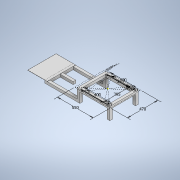
# Autodesk Inventor part: test1
Saved by Autodesk Inventor 2021 (Build 250183000, 183)
## iProperties
Created: 2023-12-08
Part Number: test1
Material: Generic
Document SubType Name: Modeling
Designer: assman
Density: 1 g/cm^3
Appearance: Default
Author: assman
Autodesk Inventor part; units mm, degrees
ref_plane "YZ Plane" through (0, 0, 0) normal (1, 0, 0) x (0, 1, 0)
ref_plane "XZ Plane" through (0, 0, 0) normal (0, 1, 0) x (-1, 0, 0)
ref_plane "XY Plane" through (0, 0, 0) normal (0, 0, 1) x (1, 0, 0)
sketch "Sketch1" plane through (0, 0, 0) normal (0, 1, 0) x (-1, 0, 0)
  line L0 (142.5, 197.5) -> (-142.5, 197.5) construction
  line L1 (-142.5, 197.5) -> (-142.5, -197.5) construction
  line L2 (-142.5, -197.5) -> (142.5, -197.5) construction
  line L3 (142.5, -197.5) -> (142.5, 197.5) construction
  line L4 (142.5, 197.5) -> (-142.5, -197.5) construction
  line L5 (-142.5, 197.5) -> (142.5, -197.5) construction
  line L6 (275, -235) -> (-275, -235) construction
  line L7 (-275, -235) -> (-275, 235) construction
  line L8 (-275, 235) -> (275, 235) construction
  line L9 (275, 235) -> (275, -235) construction
  line L10 (275, -235) -> (-275, 235) construction
  line L11 (-275, -235) -> (275, 235) construction
  line L12 (274.0052, -241.4689) -> (274.0052, -478.1407) construction
  line L13 (274.0052, -478.1407) -> (222.5538, -478.1407) construction
  line L14 (222.5538, -478.1407) -> (222.5538, -241.4689) construction
  line L15 (222.5538, -241.4689) -> (274.0052, -241.4689) construction
  line L16 (200, 212.5) -> (-200, 212.5)
  line L17 (-200, 212.5) -> (-200, 182.5)
  line L18 (-200, 182.5) -> (200, 182.5)
  line L19 (200, 182.5) -> (200, 212.5)
  line L20 (200, 212.5) -> (-200, 182.5) construction
  line L21 (-200, 212.5) -> (200, 182.5) construction
  line L22 (200, -182.5) -> (-200, -182.5)
  line L23 (-200, -182.5) -> (-200, -212.5)
  line L24 (-200, -212.5) -> (200, -212.5)
  line L25 (200, -212.5) -> (200, -182.5)
  line L26 (200, -182.5) -> (-200, -212.5) construction
  line L27 (-200, -182.5) -> (200, -212.5) construction
  circle A0 centre (142.5, 197.5) radius 4
  circle A1 centre (142.5, -197.5) radius 4
  circle A2 centre (-142.5, 197.5) radius 4
  circle A3 centre (-142.5, -197.5) radius 4
  point P0 (0, 0)
  point P1 (0, 197.5)
  point P2 (0, -197.5)
  dimension "d0" = 285
  dimension "d1" = 395
  dimension "d2" = 550
  dimension "d3" = 470
  dimension "d10" = 400
  dimension "d11" = 30
  dimension "d12" = 400
  dimension "d13" = 30
  dimension "d14" = 8
  dimension "d15" = 8
  dimension "d16" = 8
  dimension "d17" = 8
  constraints: 48 end point, 10 midpoint, 8 parallel, 4 centre point, 4 coincident, 4 horizontal, 4 perpendicular, 2 other
  measures "d0" distance of L2.end L1.end
  measures "d1" distance of L1.end L0.end
  measures "d2" distance of L7.end L8.end
  measures "d3" distance of L6.end L7.end
  measures "d10" distance of L18.end L17.end
  measures "d11" distance of L17.end L16.end
  measures "d12" distance of L24.end L23.end
  measures "d13" distance of L23.end L22.end
  measures "d14" diameter of A0
  measures "d15" diameter of A1
  measures "d16" diameter of A2
  measures "d17" diameter of A3
sketch "Sketch2" plane through (0, 0, 0) normal (0, 1, 0) x (-1, 0, 0)
  line L0 (142.5, 197.5) -> (-142.5, 197.5) construction
  line L1 (142.5, -197.5) -> (142.5, 197.5) construction
  line L2 (-142.5, -197.5) -> (142.5, -197.5) construction
  line L3 (-142.5, 197.5) -> (-142.5, -197.5) construction
  line L4 (250, 217.5) -> (-250, 217.5)
  line L5 (-250, 217.5) -> (-250, 177.5)
  line L6 (-250, 177.5) -> (250, 177.5)
  line L7 (250, 177.5) -> (250, 217.5)
  line L8 (250, 217.5) -> (-250, 177.5) construction
  line L9 (-250, 217.5) -> (250, 177.5) construction
  line L10 (250, -177.5) -> (-250, -177.5)
  line L11 (-250, -177.5) -> (-250, -217.5)
  line L12 (-250, -217.5) -> (250, -217.5)
  line L13 (250, -217.5) -> (250, -177.5)
  line L14 (250, -177.5) -> (-250, -217.5) construction
  line L15 (-250, -177.5) -> (250, -217.5) construction
  line L16 (250, 217.5) -> (210, 217.5)
  line L17 (210, 217.5) -> (210, -217.5)
  line L18 (210, -217.5) -> (250, -217.5)
  line L19 (250, -217.5) -> (250, 217.5)
  line L20 (-250, 217.5) -> (-210, 217.5)
  line L21 (-210, 217.5) -> (-210, -217.5)
  line L22 (-210, -217.5) -> (-250, -217.5)
  line L23 (-250, -217.5) -> (-250, 217.5)
  point P0 (0, 0)
  point P1 (0, 197.5)
  point P2 (0, -197.5)
  point P3 (210, -177.5)
  point P4 (-210, -177.5)
  point P5 (-210, 177.5)
  point P6 (210, 177.5)
  dimension "d4" = 500
  dimension "d5" = 40
  dimension "d6" = 500
  dimension "d7" = 40
  dimension "d8" = 40
  dimension "d9" = 40
  constraints: 40 end point, 8 parallel, 6 midpoint, 4 horizontal, 4 perpendicular, 2 point on line
  measures "d4" distance of L6.end L5.end
  measures "d5" distance of L5.end L4.end
  measures "d6" distance of L12.end L11.end
  measures "d7" distance of L11.end L10.end
  measures "d8" distance of L18.end L17.end
  measures "d9" distance of L21.end L22.end
extrude "Extrusion1" add sketch "Sketch2" against normal blind 40 contours L7 L6 L17 L4 | L17 L6 L21 L4 | L19 L10 L17 L6 | L21 L6 L5 L4 | L13 L12 L17 L10 | L21 L10 L23 L6 | L17 L12 L21 L10 | L21 L12 L11 L10
extrude "Extrusion2" add sketch "Sketch1" along normal blind 10
sketch "Sketch3" plane through (0, -40, 0) normal (0, -1, 0) x (1, 0, 0)
  line L0 (250, -217.5) -> (250, 217.5) construction
  line L1 (250, 217.5) -> (-250, 217.5) construction
  line L2 (-250, -217.5) -> (250, -217.5) construction
  line L3 (-250, 217.5) -> (-250, -217.5) construction
  line L4 (250, 217.5) -> (250, -217.5) projected
  line L5 (210, 177.5) -> (210, -177.5) projected
  line L6 (250, 217.5) -> (210, 217.5)
  line L7 (210, 217.5) -> (210, 177.5)
  line L8 (210, 177.5) -> (250, 177.5)
  line L9 (250, 177.5) -> (250, 217.5)
  line L10 (250, -217.5) -> (-250, -217.5) projected
  line L11 (210, -177.5) -> (250, -177.5)
  line L12 (250, -177.5) -> (250, -217.5)
  line L13 (250, -217.5) -> (210, -217.5)
  line L14 (210, -217.5) -> (210, -177.5)
  line L15 (-250, -217.5) -> (-210.2265, -217.5)
  line L16 (-210.2265, -217.5) -> (-210.2265, -177.5)
  line L17 (-210.2265, -177.5) -> (-250, -177.5)
  line L18 (-250, -177.5) -> (-250, -217.5)
  line L19 (-210, 177.5) -> (-210, -177.5) projected
  line L20 (-250, -217.5) -> (-250, 217.5) projected
  line L21 (-210, 177.5) -> (-250, 177.5)
  line L22 (-250, 177.5) -> (-250, 217.5)
  line L23 (-250, 217.5) -> (-210, 217.5)
  line L24 (-210, 217.5) -> (-210, 177.5)
  point P0 (0, 0)
  constraints: 32 end point, 8 parallel, 4 horizontal, 4 perpendicular, 1 point on line
extrude "Extrusion3" add sketch "Sketch3" along normal blind 150 contours L20 L23 L24 L21 | L10 L18 L17 L16 | L4 L8 L7 L6 | L4 L10 L14 L11
sketch "Sketch4" plane through (-250, 0, -217.5) normal (-1, 0, 0) x (0, 0, 1)
  line L0 (0, 0) -> (435, 0) construction
  line L1 (0, 0) -> (0, -190) construction
  line L2 (40, -190) -> (0, -190) construction
  line L3 (40, -40) -> (40, -190) construction
  line L4 (395, -40) -> (40, -40) construction
  line L5 (395, -40) -> (395, -190) construction
  line L6 (435, -190) -> (395, -190) construction
  line L7 (435, 0) -> (435, -190) construction
  line L8 (0, -40) -> (0, -190) projected
  line L9 (40, -40) -> (40, -190) projected
  line L10 (0, -190) -> (40, -190)
  line L11 (40, -190) -> (40, -150)
  line L12 (40, -150) -> (0, -150)
  line L13 (0, -150) -> (0, -190)
  line L14 (395, -40) -> (395, -190) projected
  line L15 (435, 0) -> (435, -190) projected
  line L16 (395, -190) -> (435, -190)
  line L17 (435, -190) -> (435, -150)
  line L18 (435, -150) -> (395, -150)
  line L19 (395, -150) -> (395, -190)
  point P0 (217.5, 0)
  dimension "d24" = 40
  dimension "d25" = 40
  constraints: 16 end point, 4 parallel, 2 horizontal, 2 perpendicular, 2 point on line
  measures "d24" distance of L11.end L10.end
  measures "d25" distance of L17.end L16.end
extrude "Extrusion4" add sketch "Sketch4" along normal blind 500
sketch "Sketch5" plane through (-250, -40, -177.5) normal (0, 0, 1) x (1, 0, 0)
  line L0 (0, 0) -> (39.7735, 0) construction
  line L1 (0, 0) -> (0, -110) construction
  line L2 (0, -110) -> (-500, -110) construction
  line L3 (-500, -150) -> (-500, -110) construction
  line L4 (39.7735, -150) -> (-500, -150) construction
  line L5 (39.7735, 0) -> (39.7735, -150) construction
  line L6 (0, -110) -> (-500, -110) projected
  line L7 (-500, -110) -> (-460, -110)
  line L8 (-460, -110) -> (-460, -150)
  line L9 (-460, -150) -> (-500, -150)
  line L10 (-500, -150) -> (-500, -110)
  point P0 (250, 40)
  dimension "d28" = 40
  dimension "d29" = 40
  constraints: 8 end point, 2 parallel, 1 horizontal, 1 perpendicular
  measures "d28" distance of L8.end L9.end
  measures "d29" distance of L7.end L8.end
extrude "Extrusion5" add sketch "Sketch5" along normal up to surface (355 mm away)
sketch "Sketch6" plane through (-250, -150, 217.5) normal (0, 1, 0) x (1, 0, 0)
  line L0 (0, 40) -> (0, 0) construction
  line L1 (0, 40) -> (-460, 40) construction
  line L2 (-460, 395) -> (-460, 40) construction
  line L3 (0, 395) -> (-460, 395) construction
  line L4 (0, 435) -> (0, 395) construction
  line L5 (0, 435) -> (-500, 435) construction
  line L6 (-500, 0) -> (-500, 435) construction
  line L7 (0, 0) -> (-500, 0) construction
  line L8 (-460, 0) -> (-760, 0)
  line L9 (-760, 0) -> (-760, 435)
  line L10 (-760, 435) -> (-460, 435)
  line L11 (-460, 435) -> (-460, 0)
  point P0 (250, 217.5)
  dimension "d32" = 300
  constraints: 8 end point, 2 parallel, 1 horizontal, 1 perpendicular, 1 point on line
  measures "d32" distance of L9.end L10.end
extrude "Extrusion6" add sketch "Sketch6" along normal blind 3
sketch "Sketch7" plane through (-710, -190, -177.5) normal (1, 0, 0) x (0, 0, -1)
  line L0 (-355, 0) -> (-355, 40) construction
  line L1 (0, 0) -> (-355, 0) construction
  line L2 (0, 40) -> (0, 0) construction
  line L3 (40, 40) -> (0, 40) construction
  line L4 (40, 40) -> (40, 43) construction
  line L5 (-395, 43) -> (40, 43) construction
  line L6 (-395, 40) -> (-395, 43) construction
  line L7 (-355, 40) -> (-395, 40) construction
  line L8 (-197.5, 40) -> (-157.5, 40)
  line L9 (-157.5, 40) -> (-157.5, 0)
  line L10 (-157.5, 0) -> (-197.5, 0)
  line L11 (-197.5, 0) -> (-197.5, 40)
  line L12 (-197.5, 40) -> (-157.5, 0) construction
  line L13 (-157.5, 40) -> (-197.5, 0) construction
  point P0 (-177.5, 190)
  point P1 (-177.5, 20)
  dimension "d35" = 40
  dimension "d36" = 40
  constraints: 12 end point, 2 midpoint, 2 parallel, 1 horizontal, 1 perpendicular
  measures "d35" distance of L9.end L10.end
  measures "d36" distance of L8.end L9.end
extrude "Extrusion7" add sketch "Sketch7" along normal blind 200
body "Solid1"
